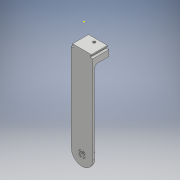
# Autodesk Inventor part: arm_segment_1_2b
Saved by Autodesk Inventor 2018 (Build 220112000, 112)
## iProperties
Created: 2018-03-21
Part Number: arm_segment_1_2b
Material: Generic
Document SubType Name: Modeling
Designer: mshaw2
Density: 1 g/cm^3
Appearance: Default
Author: mshaw2
Autodesk Inventor part; units mm, degrees
ref_plane "YZ Plane" through (0, 0, 0) normal (1, 0, 0) x (0, 1, 0)
ref_plane "XZ Plane" through (0, 0, 0) normal (0, 1, 0) x (-1, 0, 0)
ref_plane "XY Plane" through (0, 0, 0) normal (0, 0, 1) x (1, 0, 0)
sketch "Sketch1" plane through (0, 0, 0) normal (0, 1, 0) x (-1, 0, 0)
  circle A0 centre (14, -52) radius 5.5 construction
  circle A1 centre (-14, -52) radius 5.5 construction
  circle A2 centre (-4.2824, 7.9159) radius 0.75 construction
  circle A3 centre (3.4651, 8.3062) radius 0.75 construction
  circle A4 centre (6.0357, 6.6761) radius 0.75 construction
  circle A5 centre (7.9159, 4.2824) radius 0.75 construction
  circle A6 centre (8.3062, -3.4651) radius 0.75 construction
  circle A7 centre (6.6761, -6.0357) radius 0.75 construction
  circle A8 centre (4.2824, -7.9159) radius 0.75 construction
  circle A9 centre (-3.4651, -8.3062) radius 0.75 construction
  circle A10 centre (-6.0357, -6.6761) radius 0.75 construction
  circle A11 centre (-7.9159, -4.2824) radius 0.75 construction
  circle A12 centre (-6.6761, 6.0357) radius 0.75 construction
  circle A13 centre (-8.3062, 3.4651) radius 0.75 construction
  circle A14 centre (0, 0) radius 6 construction
  line L0 (28, -68) -> (28, 0) construction
  arc A15 (28, 0) -> (-28, 0) centre (0, 0) ccw construction
  line L1 (-28, 0) -> (-28, -68) construction
  line L2 (-28, -68) -> (-22, -68) construction
  line L3 (-22, -68) -> (-22, -64) construction
  line L4 (-22, -64) -> (-24.8396, -64) construction
  line L5 (-24.8396, -64) -> (-25.8396, -63) construction
  line L6 (-25.8396, -63) -> (-25.8396, -61) construction
  line L7 (-25.8396, -61) -> (-24.8396, -60) construction
  line L8 (-24.8396, -60) -> (24.8396, -60) construction
  line L9 (24.8396, -60) -> (25.8396, -61) construction
  line L10 (25.8396, -61) -> (25.8396, -63) construction
  line L11 (25.8396, -63) -> (24.8396, -64) construction
  line L12 (24.8396, -64) -> (22, -64) construction
  line L13 (22, -64) -> (22, -68) construction
  line L14 (22, -68) -> (28, -68) construction
  line L15 (0, 0) -> (0, -300) construction
  line L16 (-28.3, 0) -> (-28.3, -300) construction
  line L17 (28.3, -300) -> (28.3, 0) construction
  arc A16 (28.3, 0) -> (-28.3, 0) centre (0, 0) ccw construction
  arc A17 (-28.3, -300) -> (28.3, -300) centre (0, -300) ccw construction
  line L18 (21.7, -63.7) -> (24.7153, -63.7)
  line L19 (24.7153, -63.7) -> (25.5396, -62.8757)
  line L20 (25.5396, -62.8757) -> (25.5396, -61.1243)
  line L21 (25.5396, -61.1243) -> (24.7153, -60.3)
  line L22 (24.7153, -60.3) -> (-24.7153, -60.3)
  line L23 (-24.7153, -60.3) -> (-25.5396, -61.1243)
  line L24 (-25.5396, -61.1243) -> (-25.5396, -62.8757)
  line L25 (-25.5396, -62.8757) -> (-24.7153, -63.7)
  line L26 (-24.7153, -63.7) -> (-21.7, -63.7)
  line L27 (-21.7, -63.7) -> (-21.7, -68.3)
  line L28 (-21.7, -68.3) -> (-28.3, -68.3) construction
  line L29 (-28.3, -68.3) -> (-28.3, 0) construction
  arc A18 (28.3, 0) -> (-28.3, 0) centre (0, 0) ccw construction
  line L30 (28.3, 0) -> (28.3, -68.3) construction
  line L31 (28.3, -68.3) -> (21.7, -68.3) construction
  line L32 (21.7, -68.3) -> (21.7, -63.7)
  arc A19 (-28.3, -300) -> (28.3, -300) centre (0, -300) ccw
  line L33 (0, -150) -> (28.3, -150) construction
  circle A20 centre (-4.2824, -307.9159) radius 0.75
  circle A21 centre (3.4651, -308.3062) radius 0.75
  circle A22 centre (6.0357, -306.6761) radius 0.75
  circle A23 centre (7.9159, -304.2824) radius 0.75
  circle A24 centre (8.3062, -296.5349) radius 0.75
  circle A25 centre (6.6761, -293.9643) radius 0.75
  circle A26 centre (4.2824, -292.0841) radius 0.75
  circle A27 centre (-3.4651, -291.6938) radius 0.75
  circle A28 centre (-6.0357, -293.3239) radius 0.75
  circle A29 centre (-7.9159, -295.7176) radius 0.75
  circle A30 centre (-6.6761, -306.0357) radius 0.75
  circle A31 centre (-8.3062, -303.4651) radius 0.75
  circle A32 centre (0, -300) radius 6
  line L34 (-28.3, -300) -> (-28.3, -68.3)
  line L35 (-28.3, -68.3) -> (-21.7, -68.3)
  line L36 (21.7, -68.3) -> (28.3, -68.3)
  line L37 (28.3, -68.3) -> (28.3, -300)
  point P0 (0, -150)
  dimension "d0" = 300
  dimension "d1" = 0.3
  dimension "d2" = 150
  constraints: 78 end point, 33 centre point, 15 symmetric about line, 10 point on circle, 7 vertical, 6 horizontal, 6 tangent, 3 perpendicular, 2 equal length, 2 midpoint, 1 coincident, 82 other
  measures "d0" distance of L15.start L15.end
  measures "d1" distance between parallel lines of L12 L18
  measures "d2" distance from line of L15.end L33
extrude "Extrusion1" add sketch "Sketch1" against normal blind 5
sketch "Sketch2" plane through (0, 0, 0) normal (0, 1, 0) x (1, 0, 0)
  circle A0 centre (0, 300) radius 6 construction
  circle A1 centre (8.3062, 303.4651) radius 0.75 construction
  circle A2 centre (6.6761, 306.0357) radius 0.75 construction
  circle A3 centre (-7.9159, 304.2824) radius 0.75 construction
  circle A4 centre (-6.0357, 306.6761) radius 0.75 construction
  circle A5 centre (-3.4651, 308.3062) radius 0.75 construction
  circle A6 centre (4.2824, 307.9159) radius 0.75 construction
  circle A7 centre (3.4651, 291.6938) radius 0.75 construction
  circle A8 centre (6.0357, 293.3239) radius 0.75 construction
  circle A9 centre (7.9159, 295.7176) radius 0.75 construction
  circle A10 centre (-8.3062, 296.5349) radius 0.75 construction
  circle A11 centre (-6.6761, 293.9643) radius 0.75 construction
  circle A12 centre (-4.2824, 292.0841) radius 0.75 construction
  arc A13 (28.3, 300) -> (-28.3, 300) centre (0, 300) ccw construction
  line L0 (-28.3, 300) -> (-28.3, 68.3) construction
  line L1 (-28.3, 68.3) -> (-21.7, 68.3) projected
  line L2 (-21.7, 68.3) -> (-21.7, 63.7) projected
  line L3 (-21.7, 63.7) -> (-24.7153, 63.7) projected
  line L4 (-24.7153, 63.7) -> (-25.5396, 62.8757) projected
  line L5 (-25.5396, 62.8757) -> (-25.5396, 61.1243) projected
  line L6 (-25.5396, 61.1243) -> (-24.7153, 60.3) projected
  line L7 (-24.7153, 60.3) -> (24.7153, 60.3) projected
  line L8 (24.7153, 60.3) -> (25.5396, 61.1243) projected
  line L9 (25.5396, 61.1243) -> (25.5396, 62.8757) projected
  line L10 (25.5396, 62.8757) -> (24.7153, 63.7) projected
  line L11 (24.7153, 63.7) -> (21.7, 63.7) projected
  line L12 (21.7, 63.7) -> (21.7, 68.3) projected
  line L13 (21.7, 68.3) -> (28.3, 68.3) projected
  line L14 (28.3, 68.3) -> (28.3, 300) construction
  line L15 (-28.3, 68.3) -> (-28.3, 300) construction
  line L16 (-28.3, 68.3) -> (-28.3, 84.3)
  line L17 (-28.3, 84.3) -> (28.3, 84.3)
  line L18 (28.3, 68.3) -> (28.3, 300) construction
  line L19 (28.3, 84.3) -> (28.3, 68.3)
  point P0 (0, 0)
  dimension "d5" = 16
  constraints: 6 end point, 2 perpendicular, 2 point on line
  measures "d5" distance of L0.end L16.end
extrude "Extrusion2" add sketch "Sketch2" along normal blind 37
sketch "Sketch3" plane through (0, 0, 0) normal (0, 1, 0) x (1, 0, 0)
  point P0 (0, 0)
sketch "Sketch4" plane through (0, 0, 0) normal (0, 1, 0) x (1, 0, 0)
  line L0 (-28.3, 84.3) -> (28.3, 84.3) projected
  line L1 (28.3, 84.3) -> (28.3, 300) projected
  arc A0 (28.3, 300) -> (-28.3, 300) centre (0, 300) ccw projected
  line L2 (-28.3, 300) -> (-28.3, 84.3) projected
  circle A1 centre (0, 300) radius 6 projected
  circle A2 centre (8.3062, 303.4651) radius 0.75 projected
  circle A3 centre (6.6761, 306.0357) radius 0.75 projected
  circle A4 centre (-7.9159, 304.2824) radius 0.75 projected
  circle A5 centre (-6.0357, 306.6761) radius 0.75 projected
  circle A6 centre (-3.4651, 308.3062) radius 0.75 projected
  circle A7 centre (4.2824, 307.9159) radius 0.75 projected
  circle A8 centre (3.4651, 291.6938) radius 0.75 projected
  circle A9 centre (6.0357, 293.3239) radius 0.75 projected
  circle A10 centre (7.9159, 295.7176) radius 0.75 projected
  circle A11 centre (-8.3062, 296.5349) radius 0.75 projected
  circle A12 centre (-6.6761, 293.9643) radius 0.75 projected
  circle A13 centre (-4.2824, 292.0841) radius 0.75 projected
  circle A14 centre (0, 300) radius 13
  point P0 (0, 0)
  dimension "d8" = 26
  constraints: 1 centre point, 1 coincident
  measures "d8" diameter of A14
extrude "Extrusion3" add sketch "Sketch4" along normal blind 15.5 contours A14
sketch "Sketch5" plane through (28.3, 0, -84.3) normal (0, 0, -1) x (-1, 0, 0)
  line L0 (56.6, 0) -> (0, 0) construction
  line L1 (56.6, 0) -> (56.6, 37) construction
  line L2 (0, 37) -> (56.6, 37) construction
  line L3 (0, 0) -> (0, 37) construction
  line L4 (0, 37) -> (56.6, 37) construction
  line L5 (28.3, 37) -> (28.3, 0) construction
  point P0 (28.3, 27)
  dimension "d11" = 10
  constraints: 2 end point, 1 midpoint, 1 point on line, 1 vertical
  measures "d11" distance from line of L2 point (28.3, 27)
hole "Hole1" at (0, 27, -84.3) direction (0, 0, 1) diameter 7 end through all counterbore diameter 11 counterbore depth 8
fillet "Fillet1" radius 8 1 edges at (0, 0, -84.3)
equation "\"d2\" = 0.5 * d0"
body "Solid1"
